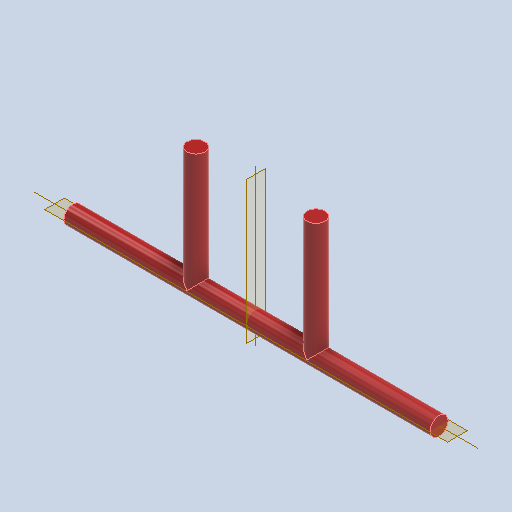
# Autodesk Inventor part: Adaptation_2_1
Saved by Autodesk Inventor 2022 (Build 260153000, 153)
## iProperties
Created: 2021-11-17
Part Number: Adaptation_2_1
Material: Generisch
Document SubType Name: Modeling
Designer: 123St
Density: 1 g/cm^3
Appearance: Rot
Mass: 0.695927 g
Surface Area: 9.44177 cm^2
Volume: 0.695927 cm^3
Author: 123St
Autodesk Inventor part; units mm, degrees
ref_plane "XY Plane" through (0, 0, 0) normal (0, 0, 1) x (1, 0, 0)
sketch "Skizze1" plane through (0, 0, 0) normal (0, 0, 1) x (1, 0, 0)
  line L0 (-30.5, 0) -> (30.5, 0)
  line L1 (30.5, 0) -> (30.5, 1.5)
  line L2 (30.5, 1.5) -> (-30.5, 1.5)
  line L3 (-30.5, 1.5) -> (-30.5, 0)
  line L4 (-42.7, 0) -> (42.7, 0) projected
  line L5 (0, 1.8) -> (0, -0.3) projected
  point P0 (0, 0)
  dimension "d0" = 61
  dimension "d1" = 1.5
  dimension "d2" = 0
  dimension "d10" = 30.5
  constraints: 8 end point, 2 parallel, 1 horizontal, 1 perpendicular
  measures "d0" distance of L1.end L2.end
  measures "d1" distance of L0.end L1.end
  measures "d2" distance between parallel lines of L4 L0
  measures "d10" distance between parallel lines of L5 L1
revolve "Umdrehung1" add sketch "Skizze1" angle 360 about axis through (0, 0, 0) along (1, 0, 0)
sketch "Skizze2" plane through (0, 0, 0) normal (0, 1, 0) x (-1, 0, 0)
  circle A0 centre (10, 0) radius 1.5
  circle A1 centre (-10, 0) radius 1.5
  point P0 (0, 0)
  dimension "d4" = 3
  dimension "d5" = 3
  dimension "d6" = 10
  dimension "d7" = 10
  constraints: 2 centre point
  measures "d4" diameter of A0
  measures "d5" diameter of A1
  measures "d6" distance of point (0, 0) A1.centre
  measures "d7" distance of point (0, 0) A0.centre
extrude "Extrusion1" add sketch "Skizze2" along normal blind 20
